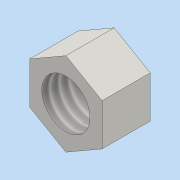
# Autodesk Inventor part: Nakrętka trapezowa 10x17
Saved by Autodesk Inventor 2018 (Build 220112000, 112)
## iProperties
Created: 2019-02-03
Part Number: Nakrętka trapezowa 10x17
Material: Ogólny
Document SubType Name: Modeling
Designer: Dawid
Density: 1 g/cm^3
Appearance: Stal
Author: Dawid
Autodesk Inventor part; units mm, degrees
ref_plane "YZ Plane" through (0, 0, 0) normal (1, 0, 0) x (0, 1, 0)
ref_plane "XZ Plane" through (0, 0, 0) normal (0, 1, 0) x (-1, 0, 0)
ref_plane "XY Plane" through (0, 0, 0) normal (0, 0, 1) x (1, 0, 0)
sketch "Szkic1" plane through (0, 0, 0) normal (0, 1, 0) x (-1, 0, 0)
  circle A0 centre (0, 0) radius 5
  line L0 (7.5, 0) -> (5, 0)
  line L1 (7.5, -4.3301) -> (0, -8.6603)
  line L2 (0, -8.6603) -> (-7.5, -4.3301)
  line L3 (-7.5, -4.3301) -> (-7.5, 4.3301)
  line L4 (-7.5, 4.3301) -> (0, 8.6603)
  line L5 (0, 8.6603) -> (7.5, 4.3301)
  line L6 (7.5, 4.3301) -> (7.5, -4.3301)
  constraints: 14 end point, 1 coincident, 1 horizontal alignment, 1 midpoint, 15 other
extrude "Wyciągnięcie proste1" add sketch "Szkic1" along normal blind 10
thread "Gwint1" size "TR10x2" class "7H" standard "ISO Metric Trapezoidal Threads" full length
